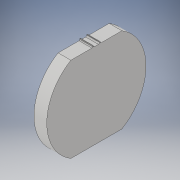
# Autodesk Inventor part: end cap
Saved by Autodesk Inventor 2017 (Build 210142000, 142)
## iProperties
Created: 2018-03-04
Part Number: end cap
Material: Generic
Document SubType Name: Modeling
Designer: Braxton
Density: 1 g/cm^3
Appearance: Default
Author: Braxton
Autodesk Inventor part; units mm, degrees
ref_plane "YZ Plane" through (0, 0, 0) normal (1, 0, 0) x (0, 1, 0)
ref_plane "XZ Plane" through (0, 0, 0) normal (0, 1, 0) x (-1, 0, 0)
ref_plane "XY Plane" through (0, 0, 0) normal (0, 0, 1) x (1, 0, 0)
sketch "Sketch1" plane through (0, 0, 0) normal (1, 0, 0) x (0, 1, 0)
  arc A0 (86.2542, -7.4083) -> (84.6667, -8.9958) centre (86.2542, -8.9958) ccw
  line L0 (87.8622, -7.4083) -> (86.2542, -7.4083)
  line L1 (87.8622, -6.35) -> (86.9132, -6.35)
  line L2 (87.8622, -7.4083) -> (87.8622, -6.35)
  arc A1 (84.6667, -4.0844) -> (86.9132, -6.35) centre (86.9324, -4.0844) ccw
  line L3 (84.6873, -6.3294) -> (87.8622, -3.1545) construction
  arc A2 (87.8622, -6.35) -> (84.6667, -3.1545) centre (84.6873, -6.3294) ccw construction
  line L4 (84.6667, -4.0844) -> (84.6667, 0)
  line L5 (87.8622, -6.35) -> (87.8622, 0) construction
  line L6 (84.6667, 0) -> (87.8622, 0) construction
  line L7 (84.6667, 8.9958) -> (84.6667, -8.9958) construction
  line L8 (84.6667, -8.9958) -> (84.6667, -50.8)
  line L9 (87.8622, 7.4083) -> (86.2542, 7.4083)
  arc A3 (84.6667, 8.9958) -> (86.2542, 7.4083) centre (86.2542, 8.9958) ccw
  line L10 (84.6873, 6.3294) -> (87.8622, 3.1545) construction
  arc A4 (84.6667, 3.1545) -> (87.8622, 6.35) centre (84.6873, 6.3294) ccw construction
  line L11 (87.8622, 6.35) -> (86.9132, 6.35)
  line L12 (87.8622, 6.35) -> (87.8622, 0) construction
  arc A5 (86.9132, 6.35) -> (84.6667, 4.0844) centre (86.9324, 4.0844) ccw
  line L13 (87.8622, 6.35) -> (87.8622, 7.4083)
  line L14 (84.6667, 8.9958) -> (84.6667, 50.8)
  line L15 (84.6667, 4.0844) -> (84.6667, 0)
  arc A6 (-84.6667, -50.8) -> (84.6667, -50.8) centre (0, 0) ccw
  arc A7 (84.6667, 50.8) -> (-84.6667, 50.8) centre (0, 0) ccw
  line L16 (-84.6667, 50.8) -> (-84.6667, -50.8)
  dimension "d85" = 101.6
  dimension "d86" = 14.8167
  dimension "d87" = 98.7374
  dimension "d88" = 98.7374
  dimension "d89" = 43.3917
  dimension "d90" = 1.5875
  dimension "d91" = 1.5875
  dimension "d92" = 41.8042
  dimension "d93" = 6.35
  dimension "d94" = 3.175
  dimension "d95" = 2.2657
  dimension "d96" = 2.2466
  dimension "d97" = 45
  dimension "d98" = 84.6667
  constraints: 34 end point, 19 point on circle, 8 centre point, 7 symmetric about line, 6 point on line, 5 collinear, 4 perpendicular, 3 coincident, 3 equal length, 2 tangent, 1 equal radius, 1 parallel, 1 vertical, 3 other
  measures "d85" distance of L14.end L8.end
  measures "d86" distance of L13.end L2.start
  measures "d87" radius of A7
  measures "d88" radius of A6
  measures "d89" distance from line of L14.end L9
  measures "d90" distance from line of L8.start L0
  measures "d91" radius of A0
  measures "d92" distance of L8.start L8.end
  measures "d93" distance of L6.end L11.start
  measures "d94" distance of L11.start L10.start
  measures "d95" radius of A5
  measures "d96" horizontal distance of L15.start L11.end
  measures "d97" angle of L12 L10
  measures "d98" distance from line of L16 point (0, 0)
extrude "connection" add sketch "Sketch1" along normal blind 25.4
equation "\"d88\" = d87"
equation "\"d90\" = 0.5 * d99"
equation "\"d99\" = 3.175"
body "Solid2"
